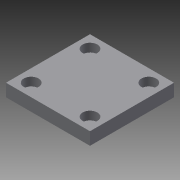
# Autodesk Inventor part: Block
Saved by Autodesk Inventor 2016 (Build 200138000, 138)
## iProperties
Created: 2014-03-06
Part Number: Block
Material: Generic
Document SubType Name: Modeling
Designer: John
Density: 1 g/cm^3
Appearance: Default
Author: John
Autodesk Inventor part; units mm, degrees
ref_plane "YZ Plane" through (0, 0, 0) normal (1, 0, 0) x (0, 1, 0)
ref_plane "XZ Plane" through (0, 0, 0) normal (0, 1, 0) x (-1, 0, 0)
ref_plane "XY Plane" through (0, 0, 0) normal (0, 0, 1) x (1, 0, 0)
sketch "Sketch1" plane through (0, 0, 0) normal (0, 1, 0) x (-1, 0, 0)
  line L0 (0, 0) -> (-63.5, 0)
  line L1 (-63.5, 0) -> (-63.5, -63.5)
  line L2 (-63.5, -63.5) -> (0, -63.5)
  line L3 (0, -63.5) -> (0, 0)
  dimension "d0" = 63.5
  dimension "d1" = 63.5
  constraints: 8 end point, 2 parallel, 1 horizontal, 1 perpendicular
  measures "d0" distance of L1.end L2.end
  measures "d1" distance of L0.end L1.end
extrude "Extrusion1" add sketch "Sketch1" along normal blind 9.525
sketch "Sketch2" plane through (0, 9.525, 0) normal (0, 1, 0) x (1, 0, 0)
  line L0 (0, 0) -> (63.5, 0) projected
  line L1 (63.5, 0) -> (63.5, 63.5) projected
  line L2 (63.5, 63.5) -> (0, 63.5) projected
  line L3 (0, 63.5) -> (0, 0) projected
  line L4 (9.525, 53.975) -> (53.975, 53.975)
  line L5 (53.975, 53.975) -> (53.975, 9.525)
  line L6 (53.975, 9.525) -> (9.525, 9.525)
  line L7 (9.525, 9.525) -> (9.525, 53.975)
  dimension "d4" = 9.525
  constraints: 8 end point, 3 other
  measures "d4" distance between parallel lines of L2 L4
hole "Hole1" at (53.975, 9.525, -9.525) at (53.975, 9.525, -53.975) at (9.525, 9.525, -53.975) at (9.525, 9.525, -9.525) direction (0, -1, 0) diameter 6.7564 end through all counterbore diameter 11.1252 counterbore depth 6.35 clearance for "Socket Head Cap Screw" size "1/4" standard "Ansi Unified Screw Threads"
equation "\"d0\" = d1"
body "Solid1"
